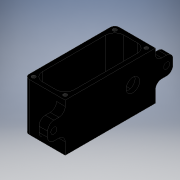
# Autodesk Inventor part: Connector Box
Saved by Autodesk Inventor 2019 (Build 230136000, 136)
## iProperties
Created: 2016-08-11
Part Number: Connector Box
Material: Aluminum 6061
Document SubType Name: Modeling
Designer: IEUser
Density: 2.7 g/cm^3
Appearance: Anodized - Black
Author: IEUser
Autodesk Inventor part; units mm, degrees
note: some values were not read from the file. Chosen so that the rebuilt part matches the saved one: direction of "Cable Exit Hole".
ref_plane "YZ Plane" through (0, 0, 0) normal (1, 0, 0) x (0, 1, 0)
ref_plane "XZ Plane" through (0, 0, 0) normal (0, 1, 0) x (-1, 0, 0)
ref_plane "XY Plane" through (0, 0, 0) normal (0, 0, 1) x (1, 0, 0)
sketch "Body Outline" plane through (0, 0, 0) normal (0, 1, 0) x (-1, 0, 0)
  line L0 (50, -22.5) -> (-50, -22.5)
  line L1 (-50, -22.5) -> (-50, 22.5)
  line L2 (-50, 22.5) -> (50, 22.5)
  line L3 (50, 22.5) -> (50, -22.5)
  point P0 (0, 0)
  dimension "d0" = 45
  dimension "d1" = 22.5
  dimension "d2" = 100
  dimension "d3" = 50
  constraints: 8 end point, 2 parallel, 1 horizontal, 1 perpendicular
  measures "d0" distance of L2.end L0.start
  measures "d1" distance from line of point (0, 0) L0
  measures "d2" distance of L0.start L0.end
  measures "d3" distance from line of point (0, 0) L3
extrude "Body" add sketch "Body Outline" along normal blind 53
shell "Shell" thickness 5 removed faces 1 at (-16.6667, 53, 7.5)
fillet "Shell Fillet" radius 10 4 edges at (-45, 29, -17.5) (45, 29, -17.5) (45, 29, 17.5) (-45, 29, 17.5)
fillet "Shell Fillet" radius 5 2 edges at (-50, 26.5, -22.5) (50, 26.5, -22.5)
sketch "Lid Fastening Hole Pattern" plane through (0, 53, 0) normal (0, 1, 0) x (1, 0, 0)
  line L0 (45, 22.5) -> (-45, 22.5) projected
  line L1 (-50, 17.5) -> (-50, -22.5) projected
  point P0 (0, 0)
  point P1 (-45, 17.5)
  point P2 (45, 17.5)
  point P3 (-45, -17.5)
  point P4 (45, -17.5)
  dimension "d115" = 5
  dimension "d116" = 5
  dimension "d119" = 90
  dimension "d122" = 35
  constraints: 1 horizontal, 1 vertical, 3 other
  measures "d115" distance from line of L0 point (-45, 17.5)
  measures "d116" distance from line of point (-45, 17.5) L1
  measures "d119" distance of point (-45, 17.5) point (45, 17.5)
  measures "d122" distance of point (-45, 17.5) point (-45, -17.5)
hole "Lid Fastening Holes" at (-45, 53, -17.5) at (45, 53, -17.5) at (-45, 53, 17.5) at (45, 53, 17.5) direction (0, -1, 0) diameter 4.134 depth 14.2 tip angle 118 thread size "M5x0.8" class "6H" standard "ISO Metric profile"
sketch "Cable Exit Hole Position" plane through (-50, 0, 22.5) normal (0, 0, 1) x (1, 0, 0)
  line L0 (100, 0) -> (0, 0) projected
  line L1 (100, 0) -> (100, 53) projected
  point P0 (50, 0)
  point P1 (75, 30)
  dimension "d167" = 30
  dimension "d168" = 25
  measures "d167" distance from line of L0 point (75, 30)
  measures "d168" distance from line of L1 point (75, 30)
hole "Cable Exit Hole" at (25, 30, 22.5) direction (0, 0, -1) diameter 15 depth 5
sketch "Flanges Outline" plane through (-50, 0, 22.5) normal (0, 0, 1) x (1, 0, 0)
  line L0 (-19.5, 40) -> (0, 40)
  line L1 (0, 40) -> (0, 20)
  line L2 (0, 20) -> (-19.5, 20)
  line L3 (-19.5, 20) -> (-19.5, 40)
  line L4 (100, 40) -> (119.5, 40)
  line L5 (119.5, 40) -> (119.5, 20)
  line L6 (119.5, 20) -> (100, 20)
  line L7 (100, 20) -> (100, 40)
  line L8 (0, 0) -> (0, 53) projected
  line L9 (100, 0) -> (100, 53) projected
  line L10 (100, 0) -> (0, 0) projected
  line L11 (0, 53) -> (100, 53) projected
  point P0 (50, 0)
  dimension "d176" = 0
  dimension "d177" = 0
  dimension "d178" = 19.5
  dimension "d179" = 19.5
  dimension "d180" = 20
  dimension "d181" = 20
  dimension "d182" = 13
  dimension "d183" = 13
  constraints: 16 end point, 4 parallel, 2 horizontal, 2 perpendicular
  measures "d176" distance between parallel lines of L8 L1
  measures "d177" distance between parallel lines of L9 L7
  measures "d178" distance of L1.end L2.end
  measures "d179" distance of L5.end L6.end
  measures "d180" distance between parallel lines of L10 L2
  measures "d181" distance between parallel lines of L10 L6
  measures "d182" distance between parallel lines of L11 L0
  measures "d183" distance between parallel lines of L11 L4
extrude "Flanges" add sketch "Flanges Outline" against normal blind 9.53 contours L0 L1 L2 L3 | L4 L5 L6 L7
fillet "Flanges Fillet" radius 7 8 edges at (-50, 40, 17.735) (-69.5, 40, 17.735) (-69.5, 20, 17.735) (-50, 20, 17.735) (50, 40, 17.735) (69.5, 40, 17.735) (69.5, 20, 17.735) (50, 20, 17.735)
sketch "Box Fastening Hole Pattern" plane through (-50, 0, 12.97) normal (0, 0, -1) x (-1, 0, 0)
  line L0 (0, 0) -> (0, 53) projected
  line L1 (-5, 0) -> (-95, 0) projected
  point P0 (-50, 0)
  point P1 (12.5, 30)
  point P2 (-112.5, 30)
  dimension "d187" = 12.5
  dimension "d188" = 30
  dimension "d191" = 125
  constraints: 1 horizontal, 1 other
  measures "d187" distance from line of point (12.5, 30) L0
  measures "d188" distance from line of point (12.5, 30) L1
  measures "d191" distance of point (12.5, 30) point (-112.5, 30)
hole "Box Fastening Holes" at (-62.5, 30, 12.97) at (62.5, 30, 12.97) direction (0, 0, 1) diameter 6.7 end through all
equation "\"d1\" = 0.5 * d0"
equation "\"d3\" = 0.5 * d2"
equation "\"d116\" = d115"
equation "\"d179\" = d178"
equation "\"d181\" = d180"
body "Solid1"
